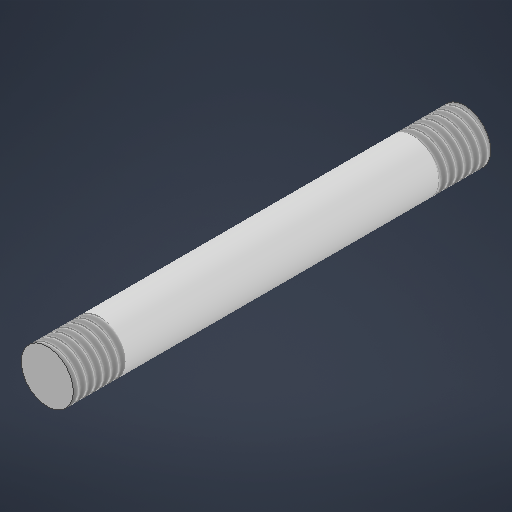
# Autodesk Inventor part: solar panel brush axle
Saved by Autodesk Inventor 2026 (Build 300175050, 175E)
## iProperties
Created: 2026-02-12
Part Number: solar panel brush axle
Material: Generic
Document SubType Name: Modeling
Designer: 268359
Density: 1 g/cm^3
Appearance: Default
Author: 268359
Autodesk Inventor part; units mm, degrees
ref_plane "YZ Plane" through (0, 0, 0) normal (1, 0, 0) x (0, 1, 0)
ref_plane "XZ Plane" through (0, 0, 0) normal (0, 1, 0) x (-1, 0, 0)
ref_plane "XY Plane" through (0, 0, 0) normal (0, 0, 1) x (1, 0, 0)
sketch "Sketch1" plane through (0, 0, 0) normal (0, 0, 1) x (1, 0, 0)
  circle A0 centre (0, 0) radius 6.35
  dimension "d0" = 12.7
  constraints: 1 centre point, 1 coincident
  measures "d0" diameter of A0
extrude "Extrusion1" add sketch "Sketch1" along normal blind 101.6
thread "Thread1" size "1/2-13 UNC" class "2A" standard "ANSI Unified Screw Threads" length 12.7
thread "Thread2" size "1/2-13 UNC" class "2A" standard "ANSI Unified Screw Threads" length 12.7
body "Solid1"
